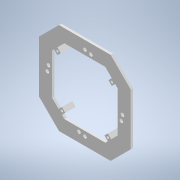
# Autodesk Inventor part: Середина
Saved by Autodesk Inventor 2021.2 (Build 252289000, 289)
## iProperties
Created: 2021-11-01
Part Number: Середина
Material: Типовые
Document SubType Name: Modeling
Designer: Kolan
Density: 1 g/cm^3
Appearance: По умолчанию
Author: Kolan
Autodesk Inventor part; units mm, degrees
ref_plane "YZ Plane" through (0, 0, 0) normal (1, 0, 0) x (0, 1, 0)
ref_plane "XZ Plane" through (0, 0, 0) normal (0, 1, 0) x (-1, 0, 0)
sketch "Эскиз1" plane through (0, 0, 0) normal (0, 0, 1) x (1, 0, 0)
  line L0 (-28.678, -17.6393) -> (-17.6393, -28.678) construction
  line L1 (-17.6393, -28.678) -> (-7, -28.678) construction
  line L2 (-7, -32.678) -> (-7, -28.678) construction
  line L3 (-3, -32.678) -> (-7, -32.678) construction
  line L4 (-3, -28.678) -> (-3, -32.678) construction
  line L5 (-3, -28.678) -> (17.6393, -28.678) construction
  line L6 (17.6393, -28.678) -> (28.678, -17.6393) construction
  line L7 (28.678, -17.6393) -> (28.678, -7) construction
  line L8 (32.678, -7) -> (28.678, -7) construction
  line L9 (32.678, -3) -> (32.678, -7) construction
  line L10 (28.678, -3) -> (32.678, -3) construction
  line L11 (28.678, -3) -> (28.678, 17.6393) construction
  line L12 (28.678, 17.6393) -> (17.6393, 28.678) construction
  line L13 (17.6393, 28.678) -> (7, 28.678) construction
  line L14 (7, 32.678) -> (7, 28.678) construction
  line L15 (3, 32.678) -> (7, 32.678) construction
  line L16 (3, 28.678) -> (3, 32.678) construction
  line L17 (3, 28.678) -> (-17.6393, 28.678) construction
  line L18 (-17.6393, 28.678) -> (-28.678, 17.6393) construction
  line L19 (-28.678, 17.6393) -> (-28.678, 7) construction
  line L20 (-32.678, 7) -> (-28.678, 7) construction
  line L21 (-32.678, 3) -> (-32.678, 7) construction
  line L22 (-28.678, 3) -> (-32.678, 3) construction
  line L23 (-28.678, 3) -> (-28.678, -17.6393) construction
  line L24 (-27.678, 17.2251) -> (-17.2251, 27.678) construction
  line L25 (-17.2251, 27.678) -> (17.2251, 27.678) construction
  line L26 (17.2251, 27.678) -> (27.678, 17.2251) construction
  line L27 (27.678, 17.2251) -> (27.678, -17.2251) construction
  line L28 (27.678, -17.2251) -> (17.2251, -27.678) construction
  line L29 (17.2251, -27.678) -> (-17.2251, -27.678) construction
  line L30 (-17.2251, -27.678) -> (-27.678, -17.2251) construction
  line L31 (-27.678, -17.2251) -> (-27.678, 17.2251) construction
  line L32 (38.678, 21.7815) -> (21.7815, 38.678)
  line L33 (21.7815, 38.678) -> (-21.7815, 38.678)
  line L34 (-21.7815, 38.678) -> (-38.678, 21.7815)
  line L35 (-38.678, 21.7815) -> (-38.678, -21.7815)
  line L36 (-38.678, -21.7815) -> (-21.7815, -38.678)
  line L37 (-21.7815, -38.678) -> (21.7815, -38.678)
  line L38 (21.7815, -38.678) -> (38.678, -21.7815)
  line L39 (38.678, -21.7815) -> (38.678, 21.7815)
  line L40 (17.2251, 27.678) -> (27.678, 17.2251)
  line L41 (27.678, 17.2251) -> (27.678, -17.2251)
  line L42 (27.678, -17.2251) -> (17.2251, -27.678)
  line L43 (17.2251, -27.678) -> (-17.2251, -27.678)
  line L44 (-17.2251, -27.678) -> (-27.678, -17.2251)
  line L45 (-27.678, -17.2251) -> (-27.678, 17.2251)
  line L46 (-27.678, 17.2251) -> (-17.2251, 27.678)
  line L47 (-17.2251, 27.678) -> (17.2251, 27.678)
  circle A0 centre (30.678, -5) radius 1.5
  circle A1 centre (5, 30.678) radius 1.5
  circle A2 centre (-30.678, 5) radius 1.5
  circle A3 centre (-5, -30.678) radius 1.5
  circle A4 centre (5, 30.678) radius 1 projected
  circle A5 centre (-30.678, 5) radius 1 projected
  circle A6 centre (30.678, -5) radius 1 projected
  circle A7 centre (-5, -30.678) radius 1 projected
  point P0 (0, 0)
  dimension "d0" = 11
  dimension "d1" = 11
  dimension "d4" = 3
  dimension "d5" = 3
  dimension "d6" = 3
  dimension "d7" = 3
  constraints: 32 end point, 4 centre point, 14 other
  measures "d0" distance between parallel lines of L26 L32
  measures "d1" distance between parallel lines of L32 L40
  measures "d4" diameter of A0
  measures "d5" diameter of A1
  measures "d6" diameter of A2
  measures "d7" diameter of A3
extrude "Выдавливание2" add sketch "Эскиз1" along normal blind 2 contours L39 L38 L37 L36 L35 L34 L33 L32
sketch "Эскиз2" plane through (0, 0, 2) normal (0, 0, 1) x (1, 0, 0)
  line L0 (21.7815, 38.678) -> (-21.7815, 38.678) construction
  line L1 (-21.7815, 38.678) -> (-38.678, 21.7815) construction
  line L2 (-38.678, 21.7815) -> (-38.678, -21.7815) construction
  line L3 (-38.678, -21.7815) -> (-21.7815, -38.678) construction
  line L4 (-21.7815, -38.678) -> (21.7815, -38.678) construction
  line L5 (21.7815, -38.678) -> (38.678, -21.7815) construction
  line L6 (38.678, -21.7815) -> (38.678, 21.7815) construction
  line L7 (38.678, 21.7815) -> (21.7815, 38.678) construction
  line L8 (17.2251, 27.678) -> (27.678, 17.2251) construction
  line L9 (27.678, 17.2251) -> (27.678, -17.2251) construction
  line L10 (27.678, -17.2251) -> (17.2251, -27.678) construction
  line L11 (17.2251, -27.678) -> (-17.2251, -27.678) construction
  line L12 (-17.2251, -27.678) -> (-27.678, -17.2251) construction
  line L13 (-27.678, -17.2251) -> (-27.678, 17.2251) construction
  line L14 (-27.678, 17.2251) -> (-17.2251, 27.678) construction
  line L15 (-17.2251, 27.678) -> (17.2251, 27.678) construction
  circle A0 centre (-5, -30.678) radius 1.5 construction
  circle A1 centre (-30.678, 5) radius 1.5 construction
  circle A2 centre (5, 30.678) radius 1.5 construction
  circle A3 centre (30.678, -5) radius 1.5 construction
  line L16 (27.678, -17.2251) -> (17.2251, -27.678) projected
  line L17 (22.1749, -22.7283) -> (19.3464, -25.5567)
  line L18 (19.3464, -25.5567) -> (16.518, -22.7283)
  line L19 (16.518, -22.7283) -> (19.3464, -19.8998)
  line L20 (19.3464, -19.8998) -> (22.1749, -22.7283)
  line L21 (17.2251, -27.678) -> (-17.2251, -27.678) construction
  line L22 (0, -27.678) -> (0, 27.678) construction
  line L23 (27.678, 17.2251) -> (27.678, -17.2251) construction
  line L24 (27.678, 0) -> (-27.678, 0) construction
  line L25 (-27.678, -17.2251) -> (-27.678, 17.2251) construction
  line L26 (-22.1749, -22.7283) -> (-19.3464, -25.5567)
  line L27 (-19.3464, -25.5567) -> (-16.518, -22.7283)
  line L28 (-16.518, -22.7283) -> (-19.3464, -19.8998)
  line L29 (-19.3464, -19.8998) -> (-22.1749, -22.7283)
  line L30 (-27.678, 17.2251) -> (-17.2251, 27.678) construction
  line L31 (22.4516, -22.4516) -> (-22.4516, 22.4516) construction
  line L32 (27.678, 17.2251) -> (17.2251, 27.678) construction
  line L33 (22.7283, 22.1749) -> (25.5567, 19.3464)
  line L34 (19.8998, 19.3464) -> (22.7283, 22.1749)
  line L35 (22.7283, 16.518) -> (19.8998, 19.3464)
  line L36 (25.5567, 19.3464) -> (22.7283, 16.518)
  circle A4 centre (19.3407, -22.734) radius 1
  circle A5 centre (-19.3738, -22.7283) radius 1
  circle A6 centre (22.7283, 19.3419) radius 1
  line L37 (-23.1587, 16.0876) -> (-20.3302, 18.916)
  line L38 (-20.3302, 18.916) -> (-23.1587, 21.7444)
  line L39 (-23.1587, 21.7444) -> (-25.9871, 18.916)
  line L40 (-25.9871, 18.916) -> (-23.1587, 16.0876)
  circle A7 centre (-23.1587, 18.9654) radius 1
  point P0 (0, 0)
  dimension "d11" = 4
  dimension "d12" = 3
  dimension "d30" = 2
  dimension "d31" = 2
  dimension "d32" = 2
  dimension "d33" = 4
  dimension "d34" = 4
  dimension "d36" = 1
  dimension "d37" = 2
  constraints: 40 end point, 8 symmetric about line, 6 midpoint, 4 centre point, 4 parallel, 4 point on line, 2 perpendicular
  measures "d11" distance of L17.end L18.end
  measures "d12" distance from line of L10.end L18
  measures "d30" diameter of A4
  measures "d31" diameter of A5
  measures "d32" diameter of A6
  measures "d33" distance of L39.end L38.end
  measures "d34" distance of L38.end L37.end
  measures "d36" distance from line of L31.end L38
  measures "d37" diameter of A7
ref_plane "РабПлоскость1" through (-27.178, -27.178, -6.6792) normal (0, 0, 1) x (1, 0, 0)
extrude "Выдавливание3" add sketch "Эскиз2" against normal up to surface (8.6792 mm away)
sketch "Эскиз3" plane through (0, 0, 2) normal (0, 0, 1) x (1, 0, 0)
  circle A0 centre (-5, -30.678) radius 1.5 construction
  circle A1 centre (30.678, -5) radius 1.5 construction
  circle A2 centre (-30.678, 5) radius 1.5 construction
  circle A3 centre (5, 30.678) radius 1.5 construction
  line L0 (-17.2251, 27.678) -> (17.2251, 27.678) construction
  line L1 (0, 27.678) -> (0, -27.678) construction
  line L2 (17.2251, -27.678) -> (-17.2251, -27.678) construction
  line L3 (27.678, 17.2251) -> (27.678, -17.2251) construction
  line L4 (27.678, 0) -> (-27.678, 0) construction
  line L5 (-27.678, -17.2251) -> (-27.678, 17.2251) construction
  circle A4 centre (0, -31.678) radius 1.5
  circle A5 centre (31.678, 0) radius 1.5
  circle A6 centre (-31.678, 0) radius 1.5
  circle A7 centre (0, 31.678) radius 1.5
  point P0 (0, 0)
  dimension "d15" = 3
  dimension "d16" = 3
  dimension "d17" = 3
  dimension "d18" = 3
  dimension "d19" = 4
  dimension "d20" = 4
  dimension "d21" = 4
  dimension "d22" = 4
  constraints: 4 centre point, 4 end point, 4 midpoint
  measures "d15" diameter of A4
  measures "d16" diameter of A5
  measures "d17" diameter of A6
  measures "d18" diameter of A7
  measures "d19" distance of L1.start A7.centre
  measures "d20" distance of L4.end A6.centre
  measures "d21" distance of L4.start A5.centre
  measures "d22" distance of A4.centre L1.end
extrude "Выдавливание4" cut sketch "Эскиз3" against normal through all
